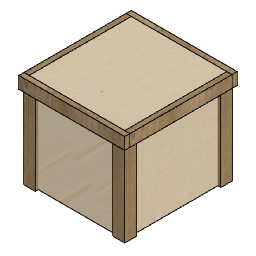
model_v1 (Autodesk Fusion 360 design; units mm, degrees)
Autodesk Fusion 360 part; units mm, degrees
note: some values were not read from the file. Chosen so that the rebuilt part matches the saved one: which bodies a step acts on.
sketch "Sketch1" plane through (0, 0, 0) normal (0, 0, 1) x (1, 0, 0)
  line L0 (0, 0) -> (28.575, 14.2875) construction
  line L1 (0, 0) -> (314.325, 0)
  line L2 (314.325, 0) -> (314.325, 338.575)
  line L3 (314.325, 338.575) -> (0, 338.575)
  line L4 (0, 338.575) -> (0, 0)
  line L5 (0, 0) -> (-19.05, -19.05) construction
  line L6 (-19.05, -19.05) -> (333.375, -19.05)
  line L7 (333.375, -19.05) -> (333.375, 357.625)
  line L8 (333.375, 357.625) -> (-19.05, 357.625)
  line L9 (-19.05, 357.625) -> (-19.05, -19.05)
  line L10 (0, 0) -> (314.325, 0)
  line L11 (314.325, 0) -> (314.325, 14.2875)
  line L12 (314.325, 14.2875) -> (0, 14.2875)
  line L13 (0, 14.2875) -> (0, 0)
  line L14 (28.575, 14.2875) -> (0, 14.2875)
  line L15 (0, 14.2875) -> (0, 338.575)
  line L16 (0, 338.575) -> (20, 338.575)
  line L17 (28.575, 324.2875) -> (28.575, 14.2875)
  line L18 (314.325, 14.2875) -> (285.75, 14.2875)
  line L19 (234.3, 338.575) -> (314.325, 338.575)
  line L20 (314.325, 338.575) -> (314.325, 14.2875)
  line L21 (47.625, 14.2875) -> (76.2, 14.2875)
  line L22 (76.2, 14.2875) -> (76.2, 54.2875)
  line L23 (76.2, 54.2875) -> (47.625, 54.2875)
  line L24 (47.625, 54.2875) -> (47.625, 14.2875)
  line L25 (0, 338.575) -> (234.3, 338.575)
  line L26 (314.325, 324.2875) -> (0, 324.2875)
  line L27 (0, 324.2875) -> (0, 338.575)
  line L28 (285.75, 324.2875) -> (285.75, 14.2875)
  line L29 (0, 338.575) -> (-19.05, 338.575)
  line L30 (314.325, 338.575) -> (333.375, 338.575)
  line L31 (314.325, 0) -> (333.375, 0)
  line L32 (-19.05, 0) -> (0, 0)
  line L33 (95.25, 54.2875) -> (95.25, 14.2875)
  line L34 (123.825, 54.2875) -> (95.25, 54.2875)
  line L35 (123.825, 14.2875) -> (123.825, 54.2875)
  line L36 (95.25, 14.2875) -> (123.825, 14.2875)
  line L37 (142.875, 54.2875) -> (142.875, 14.2875)
  line L38 (171.45, 54.2875) -> (142.875, 54.2875)
  line L39 (171.45, 14.2875) -> (171.45, 54.2875)
  line L40 (142.875, 14.2875) -> (171.45, 14.2875)
  line L41 (190.5, 54.2875) -> (190.5, 14.2875)
  line L42 (219.075, 54.2875) -> (190.5, 54.2875)
  line L43 (219.075, 14.2875) -> (219.075, 54.2875)
  line L44 (190.5, 14.2875) -> (219.075, 14.2875)
  line L45 (238.125, 54.2875) -> (238.125, 14.2875)
  line L46 (266.7, 54.2875) -> (238.125, 54.2875)
  line L47 (266.7, 14.2875) -> (266.7, 54.2875)
  line L48 (238.125, 14.2875) -> (266.7, 14.2875)
  line L49 (47.625, 324.2875) -> (47.625, 284.2875)
  line L50 (76.2, 324.2875) -> (47.625, 324.2875)
  line L51 (76.2, 284.2875) -> (76.2, 324.2875)
  line L52 (47.625, 284.2875) -> (76.2, 284.2875)
  line L53 (95.25, 324.2875) -> (95.25, 284.2875)
  line L54 (123.825, 324.2875) -> (95.25, 324.2875)
  line L55 (123.825, 284.2875) -> (123.825, 324.2875)
  line L56 (95.25, 284.2875) -> (123.825, 284.2875)
  line L57 (142.875, 324.2875) -> (142.875, 284.2875)
  line L58 (171.45, 324.2875) -> (142.875, 324.2875)
  line L59 (171.45, 284.2875) -> (171.45, 324.2875)
  line L60 (142.875, 284.2875) -> (171.45, 284.2875)
  line L61 (190.5, 324.2875) -> (190.5, 284.2875)
  line L62 (219.075, 324.2875) -> (190.5, 324.2875)
  line L63 (219.075, 284.2875) -> (219.075, 324.2875)
  line L64 (190.5, 284.2875) -> (219.075, 284.2875)
  line L65 (238.125, 324.2875) -> (238.125, 284.2875)
  line L66 (266.7, 324.2875) -> (238.125, 324.2875)
  line L67 (266.7, 284.2875) -> (266.7, 324.2875)
  line L68 (238.125, 284.2875) -> (266.7, 284.2875)
  dimension "d7" = 28.575
  dimension "d8" = 14.2875
  dimension "d13" = 314.325
  dimension "d14" = 338.575
  dimension "d15" = 19.05
  dimension "d16" = 19.05
  dimension "d17" = 352.425
  dimension "d18" = 376.675
  dimension "d19" = 14.2875
  dimension "d20" = 314.325
  dimension "d23" = 19.05
  dimension "d24" = 28.575
  dimension "d25" = 40
  dimension "d26" = 14.2875
  dimension "d27" = 28.575
  dimension "d31" = 47.625
  dimension "d32" = 270
  constraint coincident L0.start L1.start
  constraint horizontal L1
  constraint vertical L2
  constraint horizontal L3
  constraint vertical L4
  constraint horizontal L6
  constraint vertical L7
  constraint horizontal L8
  constraint vertical L9
  constraint horizontal L10
  constraint vertical L11
  constraint horizontal L12
  constraint vertical L13
  constraint horizontal L14
  constraint vertical L15
  constraint horizontal L16
  constraint vertical L17
  constraint horizontal L18
  constraint horizontal L19
  constraint vertical L20
  constraint coincident L3 L19.start
  constraint horizontal L21
  constraint vertical L22
  constraint horizontal L23
  constraint vertical L24
  constraint coincident L12 L21.start
  constraint horizontal L25
  constraint horizontal L26
  constraint vertical L27
  constraint coincident L17.start L26
  constraint coincident L2 L26.start
  constraint coincident L26 L28.start
  constraint parallel L2 L28
  constraint coincident L9 L29.end
  constraint perpendicular L9 L29
  constraint coincident L7 L30.end
  constraint perpendicular L7 L30
  constraint coincident L7 L31.end
  constraint perpendicular L7 L31
  constraint coincident L9 L32.start
  constraint perpendicular L13 L32
  measures "d7" horizontal distance of L0.start L0.end
  measures "d8" vertical distance of L0.start L0.end
  measures "d13" distance of L0.start L1.end
  measures "d14" distance of L0.start L3.end
  measures "d15" horizontal distance of L0.start L5.end
  measures "d16" vertical distance of L0.start L5.end
  measures "d17" distance of L5.end L6.end
  measures "d18" distance of L5.end L8.end
  measures "d19" distance of L0.start L12.end
  measures "d20" distance of L11.end L12.end
  measures "d23" distance of L17 L24
  measures "d24" distance of L22 L24
  measures "d25" distance of L12 L23
  measures "d26" distance of L25 L26
  measures "d27" distance of L20 L28
extrude "Extrude1" add sketch "Sketch1" along normal blind 14.2875 contours L1 L2 L4 L10 L11 L12 L13 L14 L18 L21 L36 L40 L44 L48 | L4 L12 L14 L15 L17 L26 | L2 L12 L18 L20 L26 L28 | L2 L3 L4 L15 L16 L19 L20 L25 L26 L27 L50 L54 L58 L62 L66 | L12 L17 L22 L23 L24 L26 L28 L33 L34 L35 L37 L38 L39 L41 L42 L43 L45 L46 L47 L49 L51 L52 L53 L55 L56 L57 L59 L60 L61 L63 L64 L65 L67 L68 | L12 L21 L22 L23 L24 | L12 L45 L46 L47 L48 | L26 L49 L50 L51 L52 | L26 L65 L66 L67 L68 | L12 L33 L34 L35 L36 | L12 L41 L42 L43 L44 | L26 L53 L54 L55 L56 | L26 L61 L62 L63 L64 | L12 L37 L38 L39 L40 | L26 L57 L58 L59 L60 makes body 1
extrude "Extrude2" add sketch "Sketch1" along normal blind 300 and the other way blind -14.2875 separate body contours L1 L2 L4 L10 L11 L12 L13 L14 L18 L21 L36 L40 L44 L48 | L2 L3 L4 L15 L16 L19 L20 L25 L26 L27 L50 L54 L58 L62 L66 makes body 2 at (209.55, 14.2875, 109.525) makes body 3 at (209.55, 338.575, 109.525)
extrude "Extrude3" add sketch "Sketch1" along normal blind 300 and the other way blind -14.2875 separate body contours L4 L12 L14 L15 L17 L26 | L2 L12 L18 L20 L26 L28 | L12 L21 L22 L23 L24 | L12 L45 L46 L47 L48 | L26 L49 L50 L51 L52 | L26 L65 L66 L67 L68 | L12 L33 L34 L35 L36 | L12 L41 L42 L43 L44 | L26 L53 L54 L55 L56 | L26 L61 L62 L63 L64 | L12 L37 L38 L39 L40 | L26 L57 L58 L59 L60 makes body 4 at (142.875, 40.9542, 204.7625) makes body 5 at (266.7, 297.6208, 204.7625) makes body 6 at (76.2, 297.6208, 204.7625) makes body 7 at (123.825, 297.6208, 204.7625) makes body 8 at (285.75, 117.6208, 204.7625) makes body 9 at (95.25, 40.9542, 204.7625) makes body 10 at (190.5, 40.9542, 204.7625) makes body 11 at (219.075, 297.6208, 204.7625) makes body 12 at (0, 220.9542, 109.525) makes body 13 at (171.45, 297.6208, 204.7625) makes body 14 at (238.125, 40.9542, 204.7625) makes body 15 at (47.625, 40.9542, 204.7625)
copy_body "CutPasteBodies1" bodies 1 6 7 11 8 9 10 12 2 4 3 5 13 14 15 removing the originals makes body 16 makes body 17 makes body 18 makes body 19 makes body 20 makes body 21 makes body 22 makes body 23 makes body 24 makes body 25 makes body 26 makes body 27 makes body 28 makes body 29 makes body 30 in component "foam"
extrude "Extrude1'" add sketch "Sketch1" along normal blind 310 and the other way blind 19.05 separate body contours L1 L6 L7 L9 L10 L31 L32 | L3 L7 L8 L9 L16 L19 L25 L29 L30 makes body 31 at (98.425, 0, 200.3167) makes body 32 at (215.9, 357.625, 200.3167) in component "foam"
extrude "Extrude4" add sketch "Sketch1" along normal blind 310 and the other way blind 19.05 separate body contours L4 L9 L13 L15 L27 L29 L32 | L2 L7 L11 L20 L30 L31 makes body 33 at (0, 225.7167, 90.6333) makes body 34 at (333.375, 225.7167, 200.3167)
copy_body "CutPasteBodies1'" bodies 31 32 removing the originals makes body 35 makes body 36
extrude "Extrude5" add sketch "Sketch1" against normal blind 19.05 separate body contours L1 L2 L4 L10 L11 L12 L13 L14 L18 L21 L36 L40 L44 L48 | L4 L12 L14 L15 L17 L26 | L2 L12 L18 L20 L26 L28 | L2 L3 L4 L15 L16 L19 L20 L25 L26 L27 L50 L54 L58 L62 L66 | L12 L17 L22 L23 L24 L26 L28 L33 L34 L35 L37 L38 L39 L41 L42 L43 L45 L46 L47 L49 L51 L52 L53 L55 L56 L57 L59 L60 L61 L63 L64 L65 L67 L68 | L12 L21 L22 L23 L24 | L12 L45 L46 L47 L48 | L26 L49 L50 L51 L52 | L26 L65 L66 L67 L68 | L12 L33 L34 L35 L36 | L12 L41 L42 L43 L44 | L26 L53 L54 L55 L56 | L26 L61 L62 L63 L64 | L12 L37 L38 L39 L40 | L26 L57 L58 L59 L60 makes body 37
copy_body "CutPasteBodies1''" bodies 33 34 36 37 35 removing the originals makes body 38 makes body 39 makes body 40 makes body 41 makes body 42 in component "box"
extrude "Extrude6" add sketch "Sketch1" along normal blind 329.05 and the other way blind -310 separate body makes body 43
sketch "Sketch2" plane through (0, 0, 329.05) normal (0, 0, 1) x (-1, 0, 0)
  line L0 (19.05, -357.625) -> (19.05, 19.05)
  line L1 (19.05, 19.05) -> (-333.375, 19.05)
  line L2 (-333.375, 19.05) -> (-333.375, -357.625)
  line L3 (-333.375, -357.625) -> (19.05, -357.625)
  line L4 (19.05, 19.05) -> (38.1, 38.1) construction
  line L5 (19.05, -357.625) -> (38.1, -376.675) construction
  line L6 (-333.375, -357.625) -> (-352.425, -376.675) construction
  line L7 (-333.375, 19.05) -> (-352.425, 38.1) construction
  line L8 (38.1, 38.1) -> (-352.425, 38.1)
  line L9 (-352.425, 19.05) -> (-352.425, 38.1)
  line L10 (-352.425, 19.05) -> (-333.375, 19.05)
  line L11 (38.1, 38.1) -> (38.1, 19.05)
  line L12 (38.1, 19.05) -> (19.05, 19.05)
  line L13 (19.05, 19.05) -> (-333.375, 19.05)
  line L14 (38.1, 19.05) -> (38.1, -357.625)
  line L15 (38.1, -357.625) -> (19.05, -357.625)
  line L16 (19.05, 19.05) -> (19.05, -357.625)
  line L17 (38.1, -357.625) -> (38.1, -376.675)
  line L18 (-352.425, -376.675) -> (38.1, -376.675)
  line L19 (-352.425, -376.675) -> (-352.425, -357.625)
  line L20 (-352.425, -357.625) -> (38.1, -357.625)
  line L21 (-352.425, -357.625) -> (-352.425, 19.05)
  line L22 (-333.375, 19.05) -> (-333.375, -357.625)
  dimension "d63" = 19.05
  dimension "d64" = 19.05
  dimension "d66" = 19.05
  dimension "d67" = 19.05
  dimension "d68" = 19.05
  dimension "d69" = 19.05
  dimension "d70" = 19.05
  dimension "d71" = 19.05
  constraint coincident L0.end L1.start
  constraint coincident L0.start L3.end
  constraint coincident L2.end L3.start
  constraint coincident L1.end L2.start
  constraint perpendicular L8 L9
  constraint vertical L11
  constraint horizontal L12
  constraint horizontal L10
  constraint vertical L14
  constraint horizontal L15
  constraint perpendicular L17 L20
  constraint vertical L19
  measures "d63" vertical distance of L0.end L4.end
  measures "d64" horizontal distance of L0.end L4.end
  measures "d66" vertical distance of L1.end L7.end
  measures "d67" horizontal distance of L1.end L7.end
  measures "d68" horizontal distance of L2.end L6.end
  measures "d69" vertical distance of L2.end L6.end
  measures "d70" vertical distance of L0.start L5.end
  measures "d71" horizontal distance of L0.start L5.end
extrude "Extrude7" add sketch "Sketch2" against normal blind 44.45 separate body contours L3 L15 L17 L18 L19 L20 | L1 L8 L9 L10 L11 L12 L13 makes body 44 at (92.075, 357.625, 314.2333) makes body 45 at (92.075, -19.05, 314.2333)
extrude "Extrude8" add sketch "Sketch2" against normal blind 44.45 separate body contours L0 L12 L14 L15 L16 L20 | L2 L10 L20 L21 L22 makes body 46 at (-19.05, 232.0667, 314.2333) makes body 47 at (352.425, 232.0667, 314.2333)
copy_body "CutPasteBodies1'''" bodies 43 45 44 46 47 removing the originals makes body 48 makes body 49 makes body 50 makes body 51 makes body 52 in component "lid"
sketch "Sketch3" plane through (0, 0, 0) normal (0, 0, 1) x (1, 0, 0)
  line L0 (0, 0) -> (14.2875, 14.2875) construction
  line L1 (14.2875, 14.2875) -> (300.0375, 14.2875)
  line L2 (300.0375, 14.2875) -> (300.0375, 324.2875)
  line L3 (300.0375, 324.2875) -> (14.2875, 324.2875)
  line L4 (14.2875, 324.2875) -> (14.2875, 14.2875)
  line L5 (300.0375, 14.2875) -> (344.4875, 14.2875)
  line L6 (344.4875, 14.2875) -> (344.4875, -30.1625)
  line L7 (344.4875, -30.1625) -> (300.0375, -30.1625)
  line L8 (300.0375, -30.1625) -> (300.0375, 14.2875)
  line L9 (14.2875, 14.2875) -> (-30.1625, 14.2875)
  line L10 (-30.1625, 14.2875) -> (-30.1625, -30.1625)
  line L11 (-30.1625, -30.1625) -> (14.2875, -30.1625)
  line L12 (14.2875, -30.1625) -> (14.2875, 14.2875)
  line L13 (14.2875, 324.2875) -> (-30.1625, 324.2875)
  line L14 (-30.1625, 324.2875) -> (-30.1625, 368.7375)
  line L15 (-30.1625, 368.7375) -> (14.2875, 368.7375)
  line L16 (14.2875, 368.7375) -> (14.2875, 324.2875)
  line L17 (300.0375, 324.2875) -> (344.4875, 324.2875)
  line L18 (344.4875, 324.2875) -> (344.4875, 368.7375)
  line L19 (344.4875, 368.7375) -> (300.0375, 368.7375)
  line L20 (300.0375, 368.7375) -> (300.0375, 324.2875)
  dimension "d79" = 14.2875
  dimension "d80" = 14.2875
  dimension "d81" = 285.75
  dimension "d82" = 310
  dimension "d83" = 44.45
  dimension "d84" = 44.45
  dimension "d85" = 44.45
  dimension "d86" = 44.45
  dimension "d87" = 44.45
  dimension "d88" = 44.45
  dimension "d89" = 44.45
  dimension "d90" = 44.45
  constraint coincident L0.start origin
  constraint horizontal L1
  constraint vertical L2
  constraint horizontal L3
  constraint vertical L4
  constraint horizontal L5
  constraint vertical L6
  constraint horizontal L7
  constraint vertical L8
  constraint horizontal L9
  constraint vertical L10
  constraint horizontal L11
  constraint vertical L12
  constraint horizontal L13
  constraint vertical L14
  constraint horizontal L15
  constraint vertical L16
  constraint horizontal L17
  constraint vertical L18
  constraint horizontal L19
  constraint vertical L20
  measures "d79" horizontal distance of L0.start L0.end
  measures "d80" vertical distance of L0.start L0.end
  measures "d81" distance of L2 L4
  measures "d82" distance of L1 L3
  measures "d83" distance of L1.end L7.end
  measures "d84" distance of L6 L8
  measures "d85" distance of L18 L20
  measures "d86" distance of L17 L19
  measures "d87" distance of L14 L16
  measures "d88" distance of L13 L15
  measures "d89" distance of L9 L11
  measures "d90" distance of L10 L12
extrude "Extrude9" add sketch "Sketch3" along normal blind 284.6 and the other way blind 19.05 separate body contours L13 L14 L15 L16 | L17 L18 L19 L20 | L5 L6 L7 L8 | L9 L10 L11 L12 makes body 53 at (300.0375, 353.9208, 82.1667) makes body 54 at (-0.5292, 324.2875, 183.3833) makes body 55 at (300.0375, -0.5292, 183.3833) makes body 56 at (14.2875, -15.3458, 82.1667)
copy_body "CutPasteBodies1''''" bodies 49 52 51 50 removing the originals makes body 57 makes body 58 makes body 59 makes body 60 in component "accents"
copy_body "CutPasteBodies2" bodies 56 54 55 53 removing the originals makes body 61 makes body 62 makes body 63 makes body 64 in component "accents"
component "foam" placed x (1, 0, 0) y (0, 1, 0) z (0, 0, 1) at (0, 0, 0)
component "box" placed x (1, 0, 0) y (0, 1, 0) z (0, 0, 1) at (0, 0, 0)
component "lid" placed x (1, 0, 0) y (0, 1, 0) z (0, 0, 1) at (0, 0, 0)
component "accents" placed x (1, 0, 0) y (0, 1, 0) z (0, 0, 1) at (0, 0, 0)
equation "panel_thickness = 3 / 4 * 1 in"
equation "panel_width = 310 mm"
equation "panel_length = 1105 mm"
equation "stock_thickness = 1 in * 3 / 4"
equation "foam_thickness = 1 in + 1 / 8 * 1 in"
equation "side_foam_thickness = foam_thickness / 2"
equation "d7 = foam_thickness"
equation "d8 = side_foam_thickness"
equation "inner_width = ( panel_count + 1 ) * foam_thickness + panel_count * panel_thickness"
equation "inner_depth = panel_width + 2 * side_foam_thickness"
equation "outer_width = inner_width + 2 * stock_thickness"
equation "outer_depth = inner_depth + 2 * stock_thickness"
equation "d13 = inner_width"
equation "d14 = inner_depth"
equation "d15 = stock_thickness"
equation "d16 = stock_thickness"
equation "d17 = outer_width"
equation "d18 = outer_depth"
equation "d19 = side_foam_thickness"
equation "d20 = inner_width"
equation "foam_overlap = 40 mm"
equation "d23 = panel_thickness"
equation "d24 = foam_thickness"
equation "d25 = foam_overlap"
equation "d26 = side_foam_thickness"
equation "d27 = foam_thickness"
equation "panel_count = 6"
equation "d29 = panel_count - 1"
equation "d31 = panel_thickness + foam_thickness"
equation "d32 = inner_depth - 2 * side_foam_thickness - foam_overlap"
equation "foam_height = 300 mm"
equation "foam_height_gap = 10 mm"
equation "outer_height = foam_height + foam_height_gap"
equation "d36 = side_foam_thickness"
equation "d38 = foam_height"
equation "d40 = -side_foam_thickness"
equation "d42 = foam_height"
equation "d44 = -side_foam_thickness"
equation "d46 = outer_height"
equation "d48 = outer_height"
equation "d50 = stock_thickness"
equation "d52 = stock_thickness"
equation "d54 = -stock_thickness"
equation "lid_overhang = 20 mm"
equation "lid_stock_thickness = 1 in * 3 / 4"
equation "column_stock_width = 1.75 in"
equation "d59 = outer_height + stock_thickness"
equation "d61 = -outer_height"
equation "d63 = lid_stock_thickness"
equation "d64 = lid_stock_thickness"
equation "lid_stock_width = 1.75 in"
equation "d66 = lid_stock_thickness"
equation "d67 = lid_stock_thickness"
equation "d68 = lid_stock_thickness"
equation "d69 = lid_stock_thickness"
equation "d70 = lid_stock_thickness"
equation "d71 = lid_stock_thickness"
equation "d72 = -lid_stock_width"
equation "d74 = -lid_stock_width"
equation "column_inset = side_foam_thickness"
equation "d79 = column_inset"
equation "d80 = column_inset"
equation "d81 = inner_width - 2 * column_inset"
equation "d82 = inner_depth - 2 * column_inset"
equation "d83 = column_stock_width"
equation "d84 = column_stock_width"
equation "d85 = column_stock_width"
equation "d86 = column_stock_width"
equation "d87 = column_stock_width"
equation "d88 = column_stock_width"
equation "d89 = column_stock_width"
equation "d90 = column_stock_width"
equation "d91 = outer_height + stock_thickness - lid_stock_width"
equation "d93 = stock_thickness"
